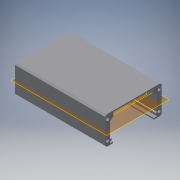
# Autodesk Inventor part: 01_Camera_Module_left_v0
Saved by Autodesk Inventor 2019.4 (Build 234330000, 330)
## iProperties
Created: 2021-09-09
Part Number: 01_Camera_Module_left_v0
Material: Generisch
Document SubType Name: Modeling
Designer: Muriel
Density: 1 g/cm^3
Appearance: Vorgabe
Mass: 9.82251 g
Surface Area: 99.5198 cm^2
Volume: 9.82251 cm^3
Author: Muriel
Autodesk Inventor part; units mm, degrees
ref_plane "Arbeitsebene6" through (-11.8704, 3.6846, 3.3435) normal (-1, 0, 0) x (0, 1, 0)
sketch "Skizze6" plane through (-11.8704, 3.6846, 3.3435) normal (-1, 0, 0) x (0, 1, 0)
  line L0 (7, 24) -> (7, 1) construction
  line L1 (7, 1) -> (8.5, 1) construction
  line L2 (8.5, 4) -> (8.5, 1) construction
  line L3 (8.5, 4) -> (11.3, 4) construction
  line L4 (11.3, 21) -> (11.3, 4) construction
  line L5 (8.5, 21) -> (11.3, 21) construction
  line L6 (8.5, 24) -> (8.5, 21) construction
  line L7 (7, 24) -> (8.5, 24) construction
  line L8 (8.5, -1) -> (8.5, 1) construction
  line L9 (7, -1) -> (8.5, -1) construction
  line L10 (7, -1) -> (7, 1) construction
  line L11 (8.5, 24) -> (8.5, 26) construction
  line L12 (7, 26) -> (8.5, 26) construction
  line L13 (7, 24) -> (7, 26) construction
  line L14 (12, 11.5) -> (8.1, 11.5)
  line L15 (3.3, 29.4) -> (12, 29.4)
  line L16 (12, 29.4) -> (12, 11.5)
  circle A0 centre (3.1, 20.5) radius 4 construction
  line L17 (7.6, 16) -> (7.6, 25) construction
  line L18 (7.6, 25) -> (-1.4, 25) construction
  line L19 (-1.4, 25) -> (-1.4, 16) construction
  line L20 (-1.4, 16) -> (7.6, 16) construction
  line L21 (3.3, 29.4) -> (-5.8, 29.4)
  line L22 (-5.8, 29.4) -> (-5.8, 11.5)
  line L23 (-5.8, 11.5) -> (8.1, 11.5)
  line L24 (3, 15.9) -> (3, 25.1)
  line L25 (5, 4.25) -> (5, 20.75) projected
  line L26 (11.3, 21) -> (11.3, 4) construction
  line L27 (7.7, 15.9) -> (7.7, 25.1)
  line L28 (7.7, 25.1) -> (-1.5, 25.1)
  line L29 (-1.5, 25.1) -> (-1.5, 15.9)
  line L30 (-1.5, 15.9) -> (7.7, 15.9)
  line L31 (3, 15.9) -> (3, 25.1)
  circle A1 centre (3.1, 20.5) radius 4 construction
  line L32 (7.6, 16) -> (7.6, 25) construction
  line L33 (7.6, 25) -> (-1.4, 25) construction
  line L34 (-1.4, 25) -> (-1.4, 16) construction
  line L35 (-1.4, 16) -> (7.6, 16) construction
  line L36 (-0.7, -1.5) -> (8.3, -1.5) construction
  line L37 (8.5, 7.7) -> (4.1628, 7.7) construction
  line L38 (-0.9, 7.7) -> (-0.9, -1.7) construction
  line L39 (8.1, 11.5) -> (8.1, 3.997) construction
  line L40 (8.1, 11.5) -> (8.1, 11.5)
  line L41 (4.1664, 7.9123) -> (4.1628, 7.7)
  point P0 (3, 11.5)
  dimension "d42" = 0.1
  dimension "d48" = 4.3
  dimension "d52" = 17.9
  dimension "d53" = 3.9
  dimension "d54" = 8.9
  dimension "d58" = 8.9
  dimension "d160" = 17.9
  dimension "d161" = 8.9
  constraints: 36 end point, 4 horizontal, 4 parallel, 4 point on line, 2 perpendicular, 2 vertical, 8 other
  measures "d42" distance between parallel lines of L20 L30
  measures "d48" distance between parallel lines of L28 L21
  measures "d52" distance between parallel lines of L23 L21
  measures "d53" distance between parallel lines of L16 L40
  measures "d54" distance from line of L21 A1.centre
  measures "d58" distance from line of L16 A0.centre
  measures "d160" distance between parallel lines of L15 L14
  measures "d161" distance from line of L22 A1.centre
ref_plane "Arbeitsebene7" through (-14.9704, 2.9846, -22.1565) normal (-1, 0, 0) x (0, 0, 1)
extrude "Extrusion6" add sketch "Skizze6" along normal up to surface (3.1 mm away)
sketch "Skizze7" plane through (-14.9704, -2.1154, -26.0565) normal (-1, 0, 0) x (0, 0, 1)
  line L0 (4.3, 4.3) -> (13.5, 4.3) projected
  line L1 (4.3, 13.5) -> (4.3, 4.3) projected
  line L2 (13.5, 13.5) -> (4.3, 13.5) projected
  line L3 (13.5, 4.3) -> (13.5, 13.5) projected
  line L4 (17.9, 17.8) -> (17.9, 0) projected
  line L5 (0, 17.8) -> (17.9, 17.8) projected
  line L6 (0, 0) -> (0, 17.8) projected
  line L7 (17.9, 0) -> (0, 0) projected
  circle A0 centre (8.95, 8.9) radius 4 construction
  circle A1 centre (8.95, 8.9) radius 4.2
  line L8 (17.9, 17.8) -> (17.9, 0) projected
  line L9 (17.9, 0) -> (0, 0) projected
  line L10 (0, 0) -> (0, 17.8) projected
  line L11 (0, 17.8) -> (17.9, 17.8) projected
  line L12 (4.3, 13.5) -> (4.3, 4.3) projected
  line L13 (4.3, 4.3) -> (13.5, 4.3) projected
  line L14 (13.5, 4.3) -> (13.5, 13.5) projected
  line L15 (13.5, 13.5) -> (4.3, 13.5) projected
  circle A2 centre (8.9, 8.9) radius 4.6 construction
  point P0 (26.0565, 2.1154)
  dimension "d141" = 8.4
  constraints: 3 centre point, 3 tangent, 1 coincident
  measures "d141" diameter of A1
extrude "Extrusion7" add sketch "Skizze7" along normal blind 2 contours L1 L2 L3 L0 | L4 L7 L6 L5
ref_plane "Arbeitsebene8" through (34.8296, 10.6846, -20.6565) normal (1, 0, 0) x (0, 1, 0)
sketch "Skizze8" plane through (-11.8704, 3.6846, 3.3435) normal (1, 0, 0) x (0, 0, -1)
  line L0 (29.4, 12) -> (29.4, -5.8) projected
  line L1 (29.4, 12) -> (11.5, 12) projected
  line L2 (29.4, -5.8) -> (25.9, -5.8)
  line L3 (25.9, -5.8) -> (25.9, 12)
  line L4 (25.9, 12) -> (29.4, 12)
  line L5 (29.4, 12) -> (29.4, -5.8)
  line L6 (25.9, 12) -> (24.2, 12)
  line L7 (24.2, 12) -> (24.2, 8.5)
  line L8 (24.2, 8.5) -> (25.9, 8.5)
  line L9 (25.9, 8.5) -> (25.9, 12)
  line L10 (24.2, 11.6) -> (24.2, 12)
  line L11 (29.4, 12) -> (25.9, 12)
  line L12 (25.9, 12) -> (25.9, -5.8)
  line L13 (25.9, -5.8) -> (29.4, -5.8)
  line L14 (29.4, -5.8) -> (29.4, 12)
  line L15 (25.9, -3.3011) -> (25.9, -5.8)
  line L16 (25.9, -2.5511) -> (25.9, -3.3011)
  line L17 (25.9, 6) -> (24.2, 6)
  line L18 (24.2, 6) -> (24.2, 5.25)
  line L19 (24.2, 5.25) -> (25.9, 5.25)
  line L20 (25.9, 5.25) -> (25.9, 6)
  line L21 (11.5, 12) -> (24.2, 12)
  line L22 (24.2, 12) -> (24.2, 11.35)
  line L23 (24.2, 11.35) -> (11.5, 11.35)
  line L24 (11.5, 11.35) -> (11.5, 12)
  line L25 (25.9, -5.8) -> (24.2, -5.8)
  line L26 (24.2, -5.8) -> (24.2, -2.3)
  line L27 (24.2, -2.3) -> (25.9, -2.3)
  line L28 (25.9, -2.3) -> (25.9, -5.8)
  line L29 (25.9, 0.2) -> (24.2, 0.2)
  line L30 (24.2, 0.2) -> (24.2, 0.95)
  line L31 (24.2, 0.95) -> (25.9, 0.95)
  line L32 (25.9, 0.95) -> (25.9, 0.2)
  point P0 (3.3435, -3.6846)
  point P1 (23, -0.4)
  dimension "d135" = 0.75
  dimension "d136" = 0.65
  dimension "d157" = 2.5
  dimension "d162" = 1.7
  dimension "d163" = 3.5
  dimension "d164" = 3.5
  dimension "d166" = 3.5
  dimension "d167" = 0.75
  dimension "d168" = 2.5
  dimension "d184" = 0
  dimension "d185" = 0
  constraints: 62 end point, 14 parallel, 7 horizontal, 7 perpendicular, 5 point on line, 1 other
  measures "d135" distance of L18.end L17.end
  measures "d136" distance of L21.end L22.end
  measures "d157" distance between parallel lines of L8 L17
  measures "d162" distance between parallel lines of L9 L7
  measures "d163" distance between parallel lines of L0 L3
  measures "d164" distance between parallel lines of L8 L1
  measures "d166" distance of L25.end L26.end
  measures "d167" distance of L29.end L30.end
  measures "d168" distance between parallel lines of L29 L27
  measures "d184" distance between parallel lines of L18 L7
  measures "d185" distance between parallel lines of L26 L18
extrude "Extrusion8" add sketch "Skizze8" along normal blind 50
chamfer "Fase1" distance 1 angle 45 2 edges at (10.5796, 15.6846, -26.0565) (10.5796, -2.1154, -26.0565)
chamfer "Fase2" distance 1 angle 45 1 edges at (-11.8704, 6.7846, -12.5565)
sketch "Skizze11" plane through (34.8296, 1.9846, -26.0565) normal (0, 0, -1) x (-1, 0, 0)
  line L0 (49.8, 0.2) -> (49.8, 9.4) projected
  line L1 (47.7, 0.2) -> (47.7, 9.4) projected
  circle A0 centre (47.7, 4.8) radius 1.4
  point P0 (34.8296, -1.9846)
  dimension "d93" = 2.8
  constraints: 1 centre point, 1 midpoint
  measures "d93" diameter of A0
extrude "Extrusion10" cut sketch "Skizze11" against normal blind 10
sketch "Skizze12" plane through (-16.9704, -2.1154, -8.1565) normal (0, -1, 0) x (1, 0, 0)
  line L0 (5.1, -12.9) -> (55.1, -12.9) projected
  line L1 (5.1, -14.9) -> (55.1, -14.9) projected
  line L2 (5.1, -12.9) -> (55.1, -12.9) projected
  line L3 (5.1, -14.9) -> (5.1, -13.6) projected
  line L4 (5.1, -14.9) -> (55.1, -14.9) projected
  line L5 (55.1, -12.9) -> (55.1, -14.9) projected
  line L6 (55.1, -14.9) -> (41.1, -14.9)
  line L7 (41.1, -14.9) -> (41.1, -8.3617)
  line L8 (41.1, -8.3617) -> (55.1, -8.3617)
  line L9 (55.1, -8.3617) -> (55.1, -14.9)
  line L10 (5.1, -13.6772) -> (55.1, -13.6772) projected
  line L11 (5.1, -23.1113) -> (5.1, 13.3678) projected
  line L12 (5.1, -14.9) -> (21.1, -14.9)
  line L13 (21.1, -14.9) -> (21.1, -8.3617)
  line L14 (21.1, -8.3617) -> (5.1, -8.3617)
  line L15 (5.1, -8.3617) -> (5.1, -14.9)
  line L16 (5.1, -12.9) -> (5.1, -13.6) projected
  point P0 (16.9704, 8.1565)
  point P1 (51.8, -13.4)
  point P2 (51.8, -14.4)
  point P3 (5.1, -13.9)
  point P4 (5.1, -13.9)
  dimension "d113" = 36
  dimension "d132" = 0
  constraints: 16 end point, 4 parallel, 2 horizontal, 2 perpendicular, 1 point on line, 2 other
  measures "d113" distance between parallel lines of L7 L11
  measures "d132" distance from line of point (5.1, -14.9) L15
ref_plane "Arbeitsebene9" through (-11.8704, 12.1846, -22.6565) normal (0, 1, 0) x (0, 0, 1)
extrude "Extrusion11" cut sketch "Skizze12" against normal blind 13 contours L11 L14 L13 L0 | L0 L13 L10 L3 L11 | L7 L8 L9 L0 | L0 L5 L10 L7 | L13 L1 L3 L10 | L10 L5 L1 L7
sketch "Skizze13" plane through (38.1296, 10.1846, -23.0565) normal (1, 0, 0) x (0, 0, -1)
  circle A0 centre (1.4, -9.3) radius 0.95
  circle A1 centre (1.4, 2.5) radius 0.95
  line L0 (-0.5, 2) -> (-0.5, 0.7) projected
  line L1 (0, -12.3) -> (2, -12.3) projected
  line L2 (3, -11.3) -> (2, -12.3) projected
  line L3 (3, -11.3) -> (3, 4.5) projected
  line L4 (2, 5.5) -> (3, 4.5) projected
  line L5 (2, 5.5) -> (-14.9, 5.5) projected
  line L6 (-14.9, 5.5) -> (-14.9, 4.85) projected
  line L7 (-14.9, 4.85) -> (-2.2, 4.85) projected
  line L8 (-2.2, 4.85) -> (-2.2, 2) projected
  line L9 (-2.2, 2) -> (-0.5, 2) projected
  line L10 (0, 0.7) -> (0, -12.3) projected
  line L11 (-0.5, 0.7) -> (0, 0.7) projected
  dimension "d182" = 3
  dimension "d183" = 3
  dimension "d190" = 1.9
  dimension "d191" = 1.9
  constraints: 2 centre point
  measures "d182" distance from line of A0.centre L1
  measures "d183" distance from line of A1.centre L5
  measures "d190" diameter of A0
  measures "d191" diameter of A1
extrude "Extrusion12" cut sketch "Skizze13" against normal blind 8 contours A0 | A1
chamfer "Fase4" distance 3 angle 45 2 edges at (-11.8704, 11.3846, -16.6565) (-11.8704, 2.1846, -16.6565)
ref_plane "Arbeitsebene10" through (30.8296, 14.9846, -11.9065) normal (0, 1, 0) x (0, 0, 1)
chamfer "Fase5" distance 1 angle 45 6 edges at (14.1296, 8.9346, -22.5565) (14.1296, 9.6846, -22.5565) (13.1296, 12.1846, -22.5565) (14.1296, 4.6346, -22.5565) (14.1296, 3.8846, -22.5565) (14.1296, 1.3846, -22.5565)
ref_plane "Arbeitsebene11" through (-16.9704, 6.7846, -17.1565) normal (0, 1, 0) x (1, 0, 0)
sketch "Skizze18" plane through (-16.9704, -2.1154, -26.0565) normal (-1, 0, 0) x (0, 0, 1)
  line L0 (17.9, 17.8) -> (1, 17.8) projected
  line L1 (0, 16.8) -> (0, 1) projected
  line L2 (1, 0) -> (17.9, 0) projected
  line L3 (17.9, 0) -> (17.9, 17.8) projected
  circle A0 centre (8.95, 8.9) radius 4.2 projected
  line L4 (17.9, 0) -> (17.9, 10) projected
  circle A1 centre (17.9, 5) radius 0.1
  line L5 (0, 16.8) -> (1, 17.8) projected
  line L6 (1, 0) -> (0, 1) projected
  point P0 (26.0565, 2.1154)
  dimension "d142" = 0.2
  constraints: 1 centre point, 1 midpoint
  measures "d142" diameter of A1
extrude "Extrusion17" cut sketch "Skizze18" against normal blind 10 contours A1 L3 | L3 A1
mirror "Spiegeln2" about plane through (-11.8704, 11.7846, -8.1565) normal (0, 0, 1) of "Extrusion6", "Extrusion7", "Extrusion8", "Fase1", "Fase2", "Extrusion11", "Extrusion12", "Fase4", "Fase5", "Extrusion17"
sketch "Skizze22" plane through (-16.9704, -2.1154, -26.0565) normal (-1, 0, 0) x (0, 0, 1)
  circle A0 centre (17.9, 5) radius 0.1 projected
  line L0 (35.8, 1) -> (34.8, 0) projected
  line L1 (35.8, 16.8) -> (35.8, 1) projected
  line L2 (34.8, 17.8) -> (35.8, 16.8) projected
  line L3 (1, 17.8) -> (34.8, 17.8) projected
  line L4 (0, 16.8) -> (1, 17.8) projected
  line L5 (0, 16.8) -> (0, 1) projected
  line L6 (1, 0) -> (0, 1) projected
  line L7 (1, 0) -> (34.8, 0) projected
  circle A1 centre (26.85, 8.9) radius 4.2 projected
  circle A2 centre (8.95, 8.9) radius 4.2 projected
  circle A3 centre (17.9, 8.9) radius 1.4
  point P0 (26.0565, 2.1154)
  dimension "d169" = 2.8
  constraints: 1 centre point
  measures "d169" diameter of A3
extrude "Extrusion21" cut sketch "Skizze22" against normal through all contours A3
sketch "Skizze23" plane through (38.1296, 3.6846, 3.3435) normal (1, 0, 0) x (0, 0, -1)
  line L0 (-2.9, 7.5) -> (-2.9, 7.2) projected
  line L1 (-1.2, 8.5) -> (-1.9, 8.5) projected
  line L2 (-1.2, 11.35) -> (-1.2, 8.5) projected
  line L3 (24.2, 11.35) -> (-1.2, 11.35) projected
  line L4 (24.2, 11.35) -> (24.2, 8.5) projected
  line L5 (24.2, 8.5) -> (24.9, 8.5) projected
  line L6 (25.9, 7.5) -> (24.9, 8.5) projected
  line L7 (25.9, 7.5) -> (25.9, 7.2) projected
  line L8 (26.4, -5.8) -> (28.4, -5.8) projected
  line L9 (29.4, -4.8) -> (28.4, -5.8) projected
  line L10 (29.4, -4.8) -> (29.4, 11) projected
  line L11 (28.4, 12) -> (29.4, 11) projected
  line L12 (28.4, 12) -> (-5.4, 12) projected
  line L13 (-6.4, 11) -> (-5.4, 12) projected
  line L14 (-6.4, -4.8) -> (-6.4, 11) projected
  line L15 (-5.4, -5.8) -> (-6.4, -4.8) projected
  line L16 (-3.4, -5.8) -> (-5.4, -5.8) projected
  circle A0 centre (-4.8, 9) radius 0.95 projected
  circle A1 centre (-4.8, -2.8) radius 0.95 projected
  circle A2 centre (27.8, -2.8) radius 0.95 projected
  circle A3 centre (27.8, 9) radius 0.95 projected
  line L17 (26.1, -4.1) -> (-2.9, -4.1) construction
  line L18 (-2.9, -4.1) -> (-2.9, -4.8) construction
  line L19 (-2.9, -4.8) -> (-1.2, -4.8) construction
  line L20 (-1.2, -4.8) -> (-1.2, -5.8) construction
  line L21 (-1.2, -5.8) -> (24.2, -5.8) construction
  line L22 (24.2, -5.8) -> (24.2, -4.8) construction
  line L23 (24.2, -4.8) -> (26.1, -4.8) construction
  line L24 (26.1, -4.8) -> (26.1, -4.1) construction
  line L25 (26.4, -5.8) -> (24.4, -5.8) construction
  line L26 (24.4, -5.8) -> (24.4, -4.9698) construction
  line L27 (24.4, -4.9698) -> (26.4, -4.9698) construction
  line L28 (26.4, -4.9698) -> (26.4, -5.8) construction
  line L29 (-3.4, -5.8) -> (26.4, -5.8) projected
  line L30 (26.4, -5.8) -> (24.4, -5.8)
  line L31 (24.4, -5.8) -> (24.4, -4.9698)
  line L32 (24.4, -4.9698) -> (26.4, -4.9698)
  line L33 (26.4, -4.9698) -> (26.4, -5.8)
  line L34 (25.9, -5.8) -> (25.9, 7.5) projected
  line L35 (-3.4, -5.8) -> (-1.4, -5.8)
  line L36 (-1.4, -5.8) -> (-1.4, -4.9698)
  line L37 (-1.4, -4.9698) -> (-3.4, -4.9698)
  line L38 (-3.4, -4.9698) -> (-3.4, -5.8)
  line L39 (-1.9, 8.5) -> (-2.9, 7.5) projected
  line L40 (-3.4, 7.2) -> (-2.9, 7.2) projected
  line L41 (25.9, 7.2) -> (26.4, 7.2) projected
  line L42 (26.4, 7.2) -> (26.4, -5.8) projected
  line L43 (-3.4, -5.8) -> (-3.4, 7.2) projected
  line L44 (26.4, -5.8) -> (26.4, 7.2) projected
  line L45 (26.4, -3.7) -> (25.4, -3.7)
  line L46 (25.4, -3.7) -> (25.4, -2.7)
  line L47 (25.4, -2.7) -> (26.4, -2.7)
  line L48 (26.4, -2.7) -> (26.4, -3.7)
  line L49 (-3.4, -5.8) -> (-3.4, 7.2) projected
  line L50 (-3.4, -3.7) -> (-2.4, -3.7)
  line L51 (-2.4, -3.7) -> (-2.4, -2.7)
  line L52 (-2.4, -2.7) -> (-3.4, -2.7)
  line L53 (-3.4, -2.7) -> (-3.4, -3.7)
  point P0 (3.3435, -3.6846)
  point P1 (26.4, 2.1202)
  dimension "d172" = 2
  dimension "d175" = 2
  dimension "d186" = 1
  dimension "d187" = 1
  dimension "d188" = 1
  dimension "d189" = 1
  constraints: 40 end point, 10 parallel, 5 horizontal, 5 perpendicular, 3 point on line, 2 other
  measures "d172" distance of L26.end L27.end
  measures "d175" distance of L37.end L36.end
  measures "d186" distance of L46.end L47.end
  measures "d187" distance of L45.end L46.end
  measures "d188" distance of L52.end L51.end
  measures "d189" distance of L51.end L50.end
extrude "Extrusion22" add sketch "Skizze23" against normal up to surface (50 mm away) contours L52 L51 L50 L43 | L37 L36 L29 L38 | L31 L32 L34 L29 | L34 L32 L33 L29 | L47 L42 L45 L34 | L34 L45 L46 L47
sketch "Skizze24" plane through (38.1296, 3.6846, 3.3435) normal (1, 0, 0) x (0, 0, -1)
  line L0 (-2.9, 7.5) -> (-2.9, 7.2) projected
  line L1 (-1.2, 8.5) -> (-1.9, 8.5) projected
  line L2 (-1.2, 11.35) -> (-1.2, 8.5) projected
  line L3 (24.2, 11.35) -> (-1.2, 11.35) projected
  line L4 (24.2, 11.35) -> (24.2, 8.5) projected
  line L5 (24.2, 8.5) -> (24.9, 8.5) projected
  line L6 (25.9, 7.5) -> (24.9, 8.5) projected
  line L7 (25.9, 7.5) -> (25.9, 7.2) projected
  line L8 (24.4, -5.8) -> (28.4, -5.8) projected
  line L9 (29.4, -4.8) -> (28.4, -5.8) projected
  line L10 (29.4, -4.8) -> (29.4, 11) projected
  line L11 (28.4, 12) -> (29.4, 11) projected
  line L12 (28.4, 12) -> (-5.4, 12) projected
  line L13 (-6.4, 11) -> (-5.4, 12) projected
  line L14 (-6.4, -4.8) -> (-6.4, 11) projected
  line L15 (-5.4, -5.8) -> (-6.4, -4.8) projected
  line L16 (-1.4, -5.8) -> (-5.4, -5.8) projected
  circle A0 centre (-4.8, 9) radius 0.95 projected
  circle A1 centre (-4.8, -2.8) radius 0.95 projected
  circle A2 centre (27.8, -2.8) radius 0.95 projected
  circle A3 centre (27.8, 9) radius 0.95 projected
  line L17 (26.4, -4.9698) -> (-3.4, -4.9698)
  line L18 (-3.4, -4.9698) -> (-3.4, -3.8)
  line L19 (-3.4, -3.8) -> (26.4, -3.8)
  line L20 (26.4, -3.8) -> (26.4, -4.9698)
  line L21 (-1.9, 8.5) -> (-2.9, 7.5) projected
  line L22 (-3.4, 7.2) -> (-2.9, 7.2) projected
  line L23 (25.9, 7.2) -> (26.4, 7.2) projected
  line L24 (26.4, 7.2) -> (26.4, -2.7) projected
  line L25 (-3.4, -4.9698) -> (-3.4, -3.7) projected
  line L26 (26.4, -2.7) -> (25.4, -2.7) projected
  line L27 (25.4, -2.7) -> (25.4, -3.7) projected
  line L28 (25.4, -3.7) -> (26.4, -3.7) projected
  line L29 (26.4, -3.7) -> (26.4, -4.9698) projected
  line L30 (26.4, -4.9698) -> (24.4, -4.9698) projected
  line L31 (24.4, -4.9698) -> (24.4, -5.8) projected
  line L32 (-1.4, -5.8) -> (-1.4, -4.9698) projected
  line L33 (-1.4, -4.9698) -> (-3.4, -4.9698) projected
  line L34 (-3.4, -3.7) -> (-2.4, -3.7) projected
  line L35 (-2.4, -3.7) -> (-2.4, -2.7) projected
  line L36 (-2.4, -2.7) -> (-3.4, -2.7) projected
  line L37 (-3.4, -2.7) -> (-3.4, 7.2) projected
  line L38 (24.4, -4.9698) -> (24.4, -5.8) projected
  line L39 (24.4, -4.9698) -> (-1.4, -4.9698)
  line L40 (-1.4, -4.9698) -> (-1.4, -5.8)
  line L41 (-1.4, -5.8) -> (24.4, -5.8)
  line L42 (24.4, -5.8) -> (24.4, -4.9698)
  point P0 (3.3435, -3.6846)
  constraints: 16 end point, 4 parallel, 2 horizontal, 2 perpendicular
extrude "Extrusion23" cut sketch "Skizze24" against normal up to surface (50 mm away) contours L19 L20 L17 L18 | L17 L31 L41 L32
sketch "Sketch25" plane through (-16.9704, -2.1154, -26.0565) normal (-1, 0, 0) x (0, 0, 1)
  circle A0 centre (17.9, 8.9) radius 1.4 projected
  circle A1 centre (17.9, 5) radius 0.1 projected
  line L0 (35.8, 1) -> (34.8, 0) projected
  line L1 (35.8, 16.8) -> (35.8, 1) projected
  line L2 (34.8, 17.8) -> (35.8, 16.8) projected
  line L3 (1, 17.8) -> (34.8, 17.8) projected
  line L4 (0, 16.8) -> (1, 17.8) projected
  line L5 (0, 16.8) -> (0, 1) projected
  line L6 (1, 0) -> (0, 1) projected
  line L7 (1, 0) -> (34.8, 0) projected
  circle A2 centre (26.85, 8.9) radius 4.2 projected
  circle A3 centre (8.95, 8.9) radius 4.2 projected
  point P0 (26.0565, 2.1154)
extrude "Extrusion24" add sketch "Sketch25" along normal blind 2
ref_plane "Arbeitsebene16" through (-16.9704, 6.7846, 0.8435) normal (0, -1, 0) x (1, 0, 0)
ref_plane "Arbeitsebene17" through (34.8296, 10.6846, 4.3435) normal (-1, 0, 0) x (0, 1, 0)
ref_plane "Arbeitsebene18" through (-11.8704, 12.1846, 6.3435) normal (0, -1, 0) x (0, 0, -1)
ref_plane "Arbeitsebene19" through (30.8296, 14.9846, -4.4065) normal (0, -1, 0) x (0, 0, -1)
